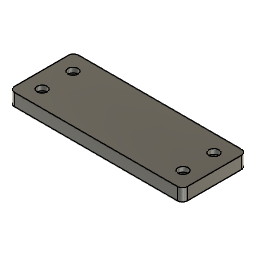
Galaxy_Front_panel (Autodesk Fusion 360 design; units mm, degrees)
Autodesk Fusion 360 part; units mm, degrees
sketch "Sketch1" plane through (0, 0, 0) normal (0, 0, 1) x (1, 0, 0)
  line L0 (66, 26) -> (-66, 26)
  line L1 (-70, 22) -> (-70, -22)
  line L2 (-66, -26) -> (66, -26)
  line L3 (70, -22) -> (70, 22)
  line L4 (70, 26) -> (-70, -26) construction
  line L5 (-70, 26) -> (70, -26) construction
  arc A0 (-70, -22) -> (-66, -26) centre (-66, -22) ccw
  arc A1 (-66, 26) -> (-70, 22) centre (-66, 22) ccw
  arc A2 (70, 22) -> (66, 26) centre (66, 22) ccw
  arc A3 (66, -26) -> (70, -22) centre (66, -22) ccw
  line L6 (-70, 26) -> (-57, 26) construction
  line L7 (-57, 26) -> (-57, 12.5) construction
  line L8 (-57, 12.5) -> (-70, 12.5) construction
  line L9 (-70, 12.5) -> (-70, 26) construction
  line L10 (70, 26) -> (57, 26) construction
  line L11 (57, 26) -> (57, 12.5) construction
  line L12 (57, 12.5) -> (70, 12.5) construction
  line L13 (70, 12.5) -> (70, 26) construction
  line L14 (-70, -26) -> (-57, -26) construction
  line L15 (-57, -26) -> (-57, -12.5) construction
  line L16 (-57, -12.5) -> (-70, -12.5) construction
  line L17 (-70, -12.5) -> (-70, -26) construction
  line L18 (70, -26) -> (57, -26) construction
  line L19 (57, -26) -> (57, -12.5) construction
  line L20 (57, -12.5) -> (70, -12.5) construction
  line L21 (70, -12.5) -> (70, -26) construction
  circle A4 centre (-57, 12.5) radius 2.2
  circle A5 centre (57, 12.5) radius 2.2
  circle A6 centre (-57, -12.5) radius 2.2
  circle A7 centre (57, -12.5) radius 2.2
  dimension "d1" = 140
  dimension "d2" = 52
  dimension "d3" = 4
  dimension "d4" = 13
  dimension "d5" = 13.5
  dimension "d6" = 13
  dimension "d7" = 13.5
  dimension "d8" = 13
  dimension "d9" = 13.5
  dimension "d10" = 13
  dimension "d11" = 13.5
  dimension "d12" = 4.4
  dimension "d13" = 4.4
  dimension "d14" = 4.4
  dimension "d15" = 4.4
  constraint horizontal L0
  constraint perpendicular L0 L1
  constraint parallel L0 L2
  constraint parallel L1 L3
  constraint coincident L4 origin
  constraint coincident L5 origin
  constraint coincident L4.end L2
  constraint coincident L4.end L1
  constraint tangent L2 A0
  constraint tangent L1 A0
  constraint coincident L5.start L1
  constraint coincident L5.start L0
  constraint tangent L1 A1
  constraint tangent L0 A1
  constraint equal A0 A1
  constraint coincident L4.start L0
  constraint coincident L4.start L3
  constraint tangent L0 A2
  constraint tangent L3 A2
  constraint equal A0 A2
  constraint coincident L5.end L3
  constraint coincident L5.end L2
  constraint tangent L3 A3
  constraint tangent L2 A3
  constraint equal A0 A3
  constraint horizontal L6
  constraint vertical L7
  constraint horizontal L8
  constraint vertical L9
  constraint horizontal L10
  constraint vertical L11
  constraint horizontal L12
  constraint vertical L13
  constraint horizontal L14
  constraint vertical L15
  constraint horizontal L16
  constraint vertical L17
  constraint horizontal L18
  constraint vertical L19
  constraint horizontal L20
  constraint vertical L21
  constraint coincident L7.end L8.start
  constraint coincident L11.end L12.start
  constraint coincident L15.end L16.start
  constraint coincident L19.end L20.start
  measures "d1" distance of L4.end L5.end
  measures "d2" distance of L5.start L4.end
  measures "d3" radius of A0
  measures "d4" distance of L5.start L6.end
  measures "d5" distance of L5.start L8.end
  measures "d6" distance of L4.start L10.end
  measures "d7" distance of L4.start L12.end
  measures "d8" distance of L4.end L14.end
  measures "d9" distance of L4.end L16.end
  measures "d10" distance of L5.end L18.end
  measures "d11" distance of L5.end L20.end
  measures "d12" diameter of A4
  measures "d13" diameter of A5
  measures "d14" diameter of A6
  measures "d15" diameter of A7
extrude "Extrude1" add sketch "Sketch1" along normal blind 10
sketch "Sketch2" plane through (0, 0, 10) normal (0, 0, 1) x (-1, 0, 0)
  circle A0 centre (57, -12.5) radius 2.2
  circle A1 centre (-57, 12.5) radius 2.2
  circle A2 centre (57, 12.5) radius 2.2
  circle A3 centre (-57, -12.5) radius 2.2
  arc A4 (-66, 26) -> (-70, 22) centre (-66, 22) ccw
  line L0 (-70, 22) -> (-70, -22)
  arc A5 (-70, -22) -> (-66, -26) centre (-66, -22) ccw
  line L1 (-66, -26) -> (66, -26)
  arc A6 (66, -26) -> (70, -22) centre (66, -22) ccw
  line L2 (70, -22) -> (70, 22)
  arc A7 (70, 22) -> (66, 26) centre (66, 22) ccw
  line L3 (66, 26) -> (-66, 26)
  circle A8 centre (57, -12.5) radius 4
  circle A9 centre (57, 12.5) radius 4
  circle A10 centre (-57, -12.5) radius 4
  circle A11 centre (-57, 12.5) radius 4
  dimension "d18" = 8
  dimension "d19" = 8
  dimension "d20" = 8
  dimension "d21" = 8
  constraint concentric A0 A8
  constraint concentric A2 A9
  constraint concentric A3 A10
  constraint concentric A1 A11
  measures "d18" diameter of A8
  measures "d19" diameter of A9
  measures "d20" diameter of A10
  measures "d21" diameter of A11
extrude "Extrude2" cut sketch "Sketch2" against normal blind 4 contours A8 | A9 | A10 | A11
